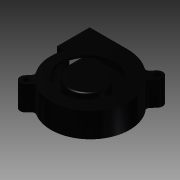
# Autodesk Inventor part: FanRadial50mm
Saved by Autodesk Inventor 2015 SP1 (Build 190203100, 203)
## iProperties
Created: 2014-12-19
Part Number: FanRadial50mm
Material: ABS Plastic
Document SubType Name: Modeling
Designer: Jack
Density: 1.06 g/cm^3
Appearance: Smooth - Black
Author: Jack
Autodesk Inventor part; units mm, degrees
ref_plane "YZ Plane" through (0, 0, 0) normal (1, 0, 0) x (0, 1, 0)
ref_plane "XZ Plane" through (0, 0, 0) normal (0, 1, 0) x (-1, 0, 0)
ref_plane "XY Plane" through (0, 0, 0) normal (0, 0, 1) x (1, 0, 0)
sketch "Sketch1" plane through (0, 0, 0) normal (0, 0, 1) x (1, 0, 0)
  line L0 (0, 0) -> (151.736327, 0) construction
  line L1 (151.736327, 0) -> (151.736327, -85.351685) construction
  line L2 (151.736327, -85.351685) -> (0, -85.351685) construction
  line L3 (0, -85.351685) -> (0, 0) construction
  circle A0 centre (92.8, -25.5) radius 1.75
  circle A1 centre (55.1, -68.251725) radius 1.75
  line L4 (47, -41) -> (47, -21)
  line L5 (47, -21) -> (70, -21)
  line L6 (47, -41) -> (51.433422, -41)
  arc A2 (51.433422, -41) -> (54.559229, -61.46466) centre (73.3, -48.131113) ccw
  arc A3 (54.429657, -63.946906) -> (54.559229, -61.46466) centre (52.929596, -62.624099) ccw
  arc A4 (61.669231, -68.413404) -> (59.099939, -68.780788) centre (60.6, -70.103595) ccw
  arc A5 (92.965603, -30.377193) -> (92.569341, -32.335578) centre (94.465664, -31.7) ccw
  arc A6 (85.567204, -25.939579) -> (88.220391, -25.628281) centre (86.72033, -24.305474) ccw
  line L7 (88.220391, -25.628281) -> (90.287399, -23.284298)
  line L8 (92.965603, -30.377193) -> (95.312601, -27.715702)
  line L9 (59.099939, -68.780788) -> (57.612601, -70.467427)
  line L10 (54.429657, -63.946906) -> (52.587399, -66.036023)
  arc A7 (52.587399, -66.036023) -> (57.612601, -70.467427) centre (55.1, -68.251725) ccw
  arc A8 (95.312601, -27.715702) -> (90.287399, -23.284298) centre (92.8, -25.5) ccw
  arc A9 (61.669231, -68.413404) -> (92.569341, -32.335578) centre (74.5, -48.131113) ccw
  arc A10 (85.567204, -25.939579) -> (70, -21) centre (70, -48) ccw
  dimension "d3" = 3.5
  dimension "d4" = 57
  dimension "d7" = 2
  dimension "d8" = 2
  dimension "d9" = 2
  dimension "d10" = 2
  dimension "d19" = 3.35
  dimension "d20" = 3.35
  dimension "d21" = 3.35
  dimension "d22" = 3.35
  dimension "d72" = 47
  dimension "d73" = 24
  dimension "d74" = 27.5
  dimension "d75" = 92.8
  dimension "d76" = 25.5
  dimension "d77" = 37.7
  dimension "d78" = 23
  dimension "d79" = 20
  dimension "d80" = 23
  dimension "d81" = 27
  dimension "d83" = 1.2
  dimension "d84" = 48
  dimension "d95" = 6.2
  dimension "d96" = 5.5
  constraints: 18 point on circle, 16 end point, 11 centre point, 10 tangent, 3 coincident, 2 parallel, 1 collinear, 1 equal radius, 1 horizontal, 1 horizontal alignment, 1 perpendicular, 1 vertical, 2 other
  measures "d3" diameter of A0
  measures "d4" distance of A0.centre A1.centre
  measures "d7" radius of A3
  measures "d8" radius of A4
  measures "d9" radius of A5
  measures "d10" radius of A6
  measures "d19" distance from line of L8 A0.centre
  measures "d20" distance from line of L7 A0.centre
  measures "d21" distance from line of A1.centre L9
  measures "d22" distance from line of A1.centre L10
  measures "d72" distance from line of point (0, 0) L4
  measures "d73" radius of A9
  measures "d74" distance from line of L4 A9.centre
  measures "d75" horizontal distance of point (0, 0) A0.centre
  measures "d76" vertical distance of A0.centre point (0, 0)
  measures "d77" horizontal distance of A0.centre A1.centre
  measures "d78" distance of L4.end L5.end
  measures "d79" distance of L4.start L4.end
  measures "d80" radius of A2
  measures "d81" radius of A10
  measures "d83" distance of A9.centre A2.centre
  measures "d84" vertical distance of L0.start A10.centre
  measures "d95" vertical distance of A0.centre A5.centre
  measures "d96" horizontal distance of A1.centre A4.centre
extrude "Extrusion1" add sketch "Sketch1" along normal blind 15
shell "Shell1" thickness 1.3 removed faces 1 at (47, -34.333333, 5)
sketch "Sketch2" plane through (0, 0, 15) normal (0, 0, 1) x (1, 0, 0)
  arc A0 (51.433422, -41) -> (54.559229, -61.46466) centre (73.3, -48.131113) ccw
  circle A1 centre (72.8, -48.131113) radius 16.5
  point P0 (0, 0)
  dimension "d100" = 33
  dimension "d101" = 0.5
  constraints: 1 centre point, 1 horizontal alignment
  measures "d100" diameter of A1
  measures "d101" distance of A0.centre A1.centre
extrude "Extrusion2" cut sketch "Sketch2" against normal up to next
sketch "Sketch3" plane through (47, -22.3, 1.3) normal (0, 0, 1) x (1, 0, 0)
  circle A0 centre (25.8, -25.831113) radius 16.5
  circle A1 centre (25.8, -25.831113) radius 12
  point P0 (-47, 22.3)
  dimension "d104" = 24
  constraints: 1 centre point, 1 coincident
  measures "d104" diameter of A1
extrude "Extrusion3" add sketch "Sketch3" along normal up to surface (13.7 mm away) contours A1
fillet "Fillet1" radius 1 1 edges at (60.8, -48.1311, 15)
body "Solid1"
